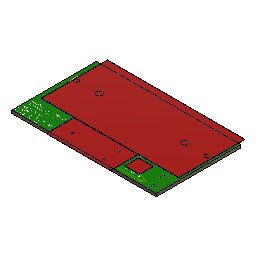
Trashcan Panda v2 v9 (Autodesk Fusion 360 archive; units mm, degrees)
design "Battery-Board"
part number: B2B-PH-SM4-TB(LF)(SN)
part number: HLC-1520A/TP
part number: 2232
Autodesk Fusion 360 part; units mm, degrees
sketch "sketch 305" plane through (0, 0, 0) normal (0, 0, 1) x (1, 0, 0)
  line L0 (0, 0) -> (77.45, 0)
  line L1 (77.45, 0) -> (77.45, 45.39)
  line L2 (77.45, 45.39) -> (0, 45.39)
  line L3 (0, 45.39) -> (0, 0)
extrude "Board" add sketch "sketch 305" along normal blind 1.57 makes body 1 in component "Board"
sketch "sketch 764" plane through (0, 0, 0) normal (0, 0, 1) x (1, 0, 0)
  line L0 (-3.975, -2.624) -> (3.975, -2.624)
  line L1 (3.975, -2.624) -> (3.975, 4.75)
  line L2 (3.975, 4.75) -> (-3.975, 4.75)
  line L3 (-3.975, 4.75) -> (-3.975, -2.624)
extrude "JST_B2B-PH-SM4-TB(LF)(SN)" add sketch "sketch 764" along normal blind 0.1 separate body makes body 2 in component "JST_B2B-PH-SM4-TB(LF)(SN)"
sketch "sketch 1034" plane through (0, 0, 0) normal (0, 0, 1) x (1, 0, 0)
  line L0 (-17.145, -7.4) -> (17.248, -7.4)
  line L1 (17.248, -7.4) -> (17.248, 7.4)
  line L2 (17.248, 7.4) -> (-17.145, 7.4)
  line L3 (-17.145, 7.4) -> (-17.145, -7.4)
extrude "HLC-1520A/TP" add sketch "sketch 1034" along normal blind 0.1 separate body makes body 3 in component "HLC-1520A/TP"
sketch "sketch 1369" plane through (0, 0, 0) normal (0, 0, 1) x (1, 0, 0)
  line L0 (-36.195, -17.78) -> (37.568, -17.78)
  line L1 (37.568, -17.78) -> (37.568, 17.78)
  line L2 (37.568, 17.78) -> (-36.195, 17.78)
  line L3 (-36.195, 17.78) -> (-36.195, -17.78)
extrude "2232" add sketch "sketch 1369" along normal blind 0.1 separate body makes body 4 in component "2232"
sketch "sketch 1173" plane through (0, 0, 0) normal (0, 0, 1) x (1, 0, 0)
  circle A0 centre (70.993, 8.763) radius 0.175
  circle A1 centre (72.644, 3.556) radius 0.175
  circle A2 centre (74.168, 3.556) radius 0.175
  circle A3 centre (72.644, 2.286) radius 0.175
  circle A4 centre (73.787, 10.668) radius 0.175
  circle A5 centre (70.993, 10.668) radius 0.175
  circle A6 centre (3.683, 31.115) radius 1.092
  circle A7 centre (73.533, 31.115) radius 1.092
  circle A8 centre (15.748, 31.115) radius 1.5875
  circle A9 centre (61.468, 31.115) radius 1.5875
  circle A10 centre (26.838, 5.715) radius 0.4
  circle A11 centre (47.838, 9.465) radius 0.4
  circle A12 centre (47.838, 1.965) radius 0.4
extrude "Extrude3" cut sketch "sketch 1173" along normal blind 1.57 bodies 1 in component "Board"
component "PCB Component" placed x (1, 0, 0) y (0, 1, 0) z (0, 0, 1) at (0, 0, 0)
component "Board" placed x (1, 0, 0) y (0, 1, 0) z (0, 0, 1) at (0, 0, 0) in component "PCB Component"
component "JST_B2B-PH-SM4-TB(LF)(SN)" placed x (1, 0, 0) y (0, 1, 0) z (0, 0, 1) at (60.198, 6.985, 1.57) in component "PCB Component"
component "HLC-1520A/TP" placed x (1, 0, 0) y (0, 1, 0) z (0, 0, 1) at (37.338, 5.715, 1.57) in component "PCB Component"
component "2232" placed x (1, 0, 0) y (0, 1, 0) z (0, 0, 1) at (38.608, 31.115, 1.57) in component "PCB Component"
named bodies: "Board", "JST_B2B-PH-SM4-TB(LF)(SN)", "HLC-1520A/TP", "2232"

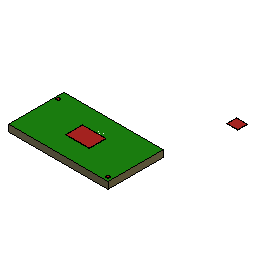
design "Sensor Breakout"
part number: FIDUCIALUFIDUCIAL
part number: 0.1uF
part number: OSHW-LOGOMINI
part number: VL53L1X
part number: 10k
part number: BM06B-SRSS-TBT(LF)(SN)
part number: LIS3DH
part number: 100k
part number: BSS215P
Autodesk Fusion 360 part; units mm, degrees
sketch "sketch 305" plane through (0, 0, 0) normal (0, 0, 1) x (1, 0, 0)
  line L0 (0, 0) -> (0, 12.7)
  line L1 (0, 12.7) -> (22.86, 12.7)
  line L2 (22.86, 12.7) -> (22.86, 0)
  line L3 (22.86, 0) -> (0, 0)
extrude "Board" add sketch "sketch 305" along normal blind 1.57 makes body 1 in component "Board"
sketch "sketch 499" plane through (0, 0, 0) normal (0, 0, 1) x (1, 0, 0)
  line L0 (-0.3175, -0.3175) -> (0.3175, -0.3175)
  line L1 (0.3175, -0.3175) -> (0.3175, 0.3175)
  line L2 (0.3175, 0.3175) -> (-0.3175, 0.3175)
  line L3 (-0.3175, 0.3175) -> (-0.3175, -0.3175)
extrude "MICRO-FIDUCIAL" add sketch "sketch 499" along normal blind 0.1 separate body makes body 2 in component "MICRO-FIDUCIAL"
sketch "sketch 634" plane through (0, 0, 0) normal (0, 0, 1) x (1, 0, 0)
  line L0 (-0.838, -0.47) -> (0.83, -0.47)
  line L1 (0.83, -0.47) -> (0.83, 0.48)
  line L2 (0.83, 0.48) -> (-0.838, 0.48)
  line L3 (-0.838, 0.48) -> (-0.838, -0.47)
extrude "0603" add sketch "sketch 634" along normal blind 0.1 separate body makes body 3 in component "0603"
sketch "sketch 769" plane through (0, 0, 0) normal (0, 0, 1) x (1, 0, 0)
  line L0 (-1.233, -0.993) -> (1.237, -0.993)
  line L1 (1.237, -0.993) -> (1.237, 1.217)
  line L2 (1.237, 1.217) -> (-1.233, 1.217)
  line L3 (-1.233, 1.217) -> (-1.233, -0.993)
extrude "OSHW-LOGO-MINI" add sketch "sketch 769" along normal blind 0.1 separate body makes body 4 in component "OSHW-LOGO-MINI"
sketch "sketch 904" plane through (0, 0, 0) normal (0, 0, 1) x (1, 0, 0)
  line L0 (-2.7, -1.941) -> (2.7, -1.941)
  line L1 (2.7, -1.941) -> (2.7, 1.9)
  line L2 (2.7, 1.9) -> (-2.7, 1.9)
  line L3 (-2.7, 1.9) -> (-2.7, -1.941)
extrude "VL53L1X" add sketch "sketch 904" along normal blind 0.1 separate body makes body 5 in component "VL53L1X"
sketch "sketch 1039" plane through (0, 0, 0) normal (0, 0, 1) x (1, 0, 0)
  line L0 (-0.838, -0.47) -> (0.83, -0.47)
  line L1 (0.83, -0.47) -> (0.83, 0.48)
  line L2 (0.83, 0.48) -> (-0.838, 0.48)
  line L3 (-0.838, 0.48) -> (-0.838, -0.47)
extrude "0603'" add sketch "sketch 1039" along normal blind 0.1 separate body makes body 6 in component "0603 (1)"
sketch "sketch 1174" plane through (0, 0, 0) normal (0, 0, 1) x (1, 0, 0)
  line L0 (-4, -3.031) -> (4, -3.031)
  line L1 (4, -3.031) -> (4, 0.7)
  line L2 (4, 0.7) -> (-4, 0.7)
  line L3 (-4, 0.7) -> (-4, -3.031)
extrude "JST_BM06B-SRSS-TB(LF)(SN)" add sketch "sketch 1174" along normal blind 0.1 separate body makes body 7 in component "JST_BM06B-SRSS-TB(LF)(SN)"
sketch "sketch 1309" plane through (0, 0, 0) normal (0, 0, 1) x (1, 0, 0)
  line L0 (-2.003, -1.5) -> (1.5, -1.5)
  line L1 (1.5, -1.5) -> (1.5, 1.5)
  line L2 (1.5, 1.5) -> (-2.003, 1.5)
  line L3 (-2.003, 1.5) -> (-2.003, -1.5)
extrude "PQFN50P300X300X100-16N" add sketch "sketch 1309" along normal blind 0.1 separate body makes body 8 in component "PQFN50P300X300X100-16N"
sketch "sketch 1444" plane through (0, 0, 0) normal (0, 0, 1) x (1, 0, 0)
  line L0 (-2.2, -1.1) -> (2.2, -1.1)
  line L1 (2.2, -1.1) -> (2.2, 1.1)
  line L2 (2.2, 1.1) -> (-2.2, 1.1)
  line L3 (-2.2, 1.1) -> (-2.2, -1.1)
extrude "C1206" add sketch "sketch 1444" along normal blind 0.1 separate body makes body 9 in component "C1206"
sketch "sketch 1579" plane through (0, 0, 0) normal (0, 0, 1) x (1, 0, 0)
  line L0 (-1.3, 0.6) -> (1.3, 0.6)
  line L1 (1.3, 0.6) -> (1.3, -0.6)
  line L2 (1.3, -0.6) -> (-1.3, -0.6)
  line L3 (-1.3, -0.6) -> (-1.3, 0.6)
extrude "0805" add sketch "sketch 1579" along normal blind 1.645 separate body makes body 10 in component "0805"
sketch "sketch 1714" plane through (0, 0, 0) normal (0, 0, 1) x (1, 0, 0)
  line L0 (-1.651, -2.642) -> (1.651, -2.642)
  line L1 (1.651, -2.642) -> (1.651, 1.321)
  line L2 (1.651, 1.321) -> (-1.651, 1.321)
  line L3 (-1.651, 1.321) -> (-1.651, -2.642)
extrude "SOT-23_3L_ONS-M" add sketch "sketch 1714" along normal blind 0.1 separate body makes body 11 in component "SOT-23_3L_ONS-M"
component "PCB Component" placed x (1, 0, 0) y (0, 1, 0) z (0, 0, 1) at (0, 0, 0)
component "Board" placed x (1, 0, 0) y (0, 1, 0) z (0, 0, 1) at (0, 0, 0) in component "PCB Component"
component "MICRO-FIDUCIAL" placed x (1, 0, 0) y (0, 1, 0) z (0, 0, 1) at (21.971, 0.889, 1.57) in component "PCB Component"
component "MICRO-FIDUCIAL" placed x (1, 0, 0) y (0, 1, 0) z (0, 0, 1) at (0.762, 10.668, 1.57) in component "PCB Component"
component "MICRO-FIDUCIAL" placed x (-1, 0, 0) y (0, 1, 0) z (0, 0, -1) at (0.762, 10.668, 0) in component "PCB Component"
component "MICRO-FIDUCIAL" placed x (-1, 0, 0) y (0, 1, 0) z (0, 0, -1) at (21.971, 0.889, 0) in component "PCB Component"
component "0603" placed x (0, -1, 0) y (-1, 0, 0) z (0, 0, -1) at (15.621, 6.35, 0) in component "PCB Component"
component "OSHW-LOGO-MINI" placed x (-1, 0, 0) y (0, 1, 0) z (0, 0, -1) at (24.638, 27.813, 0) in component "PCB Component"
component "VL53L1X" placed x (1, 0, 0) y (0, 1, 0) z (0, 0, 1) at (11.43, 6.35, 1.57) in component "PCB Component"
component "0603 (1)" placed x (0, 1, 0) y (1, 0, 0) z (0, 0, -1) at (11.303, 6.35, 0) in component "PCB Component"
component "JST_BM06B-SRSS-TB(LF)(SN)" placed x (0, -1, 0) y (-1, 0, 0) z (0, 0, -1) at (2.921, 6.35, 0) in component "PCB Component"
component "PQFN50P300X300X100-16N" placed x (0, -1, 0) y (-1, 0, 0) z (0, 0, -1) at (19.05, 6.35, 0) in component "PCB Component"
component "C1206" placed x (0, -1, 0) y (-1, 0, 0) z (0, 0, -1) at (13.462, 6.35, 0) in component "PCB Component"
component "0805" placed x (-1, 0, 0) y (0, 1, 0) z (0, 0, -1) at (6.35, 2.54, 0) in component "PCB Component"
component "SOT-23_3L_ONS-M" placed x (-1, 0, 0) y (0, 1, 0) z (0, 0, -1) at (6.35, 5.08, 0) in component "PCB Component"
named bodies: "Board", "MICRO-FIDUCIAL", "0603", "OSHW-LOGO-MINI", "VL53L1X", "JST_BM06B-SRSS-TB(LF)(SN)", "PQFN50P300X300X100-16N", "C1206", "0805", "SOT-23_3L_ONS-M"

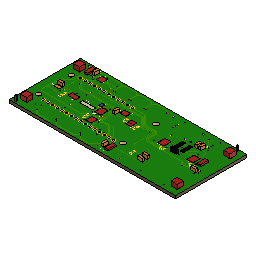
design "Carrier Board"
part number: 0.1uF
part number: D5V0L4B5TS
part number: 4.7k
part number: 100k
part number: TMP36GRTZ
part number: FIDUCIALUFIDUCIAL
part number: STAND-OFF
part number: 6V/0.5A
part number: 470uF
part number: Particle Boron / Xenon / Argon
part number: MF-SW-TACT-6MM
part number: BAT42
part number: JUMPER-SMT_2_NO_SILK
part number: 6.2V/500mW
part number: CL-SB-12B-01T
part number: BM04B-SRSS-TBT(LF)(SN)
part number: BM06B-SRSS-TBT(LF)(SN)
part number: AB1805-T3
part number: XC6215B332MR-G
part number: BSS138
part number: MB85RC64TASON8
part number: B2B-PH-SM4-TB(LF)(SN)
part number: GRM21A5C2D470JW01D
part number: BSS215P
part number: SSPT7F-7PF20-R
Autodesk Fusion 360 part; units mm, degrees
sketch "sketch 305" plane through (0, 0, 0) normal (0, 0, 1) x (1, 0, 0)
  line L0 (0, 0) -> (89.967, 0)
  line L1 (89.967, 0) -> (89.967, 38.608)
  line L2 (89.967, 38.608) -> (0, 38.608)
  line L3 (0, 38.608) -> (0, 0)
extrude "Board" add sketch "sketch 305" along normal blind 1.5723 makes body 1 in component "Board"
sketch "sketch 1247" plane through (0, 0, 0) normal (0, 0, 1) x (1, 0, 0)
  line L0 (-0.3, -0.6) -> (0.3, -0.6)
  line L1 (0.3, -0.6) -> (0.3, 0.6)
  line L2 (0.3, 0.6) -> (-0.3, 0.6)
  line L3 (-0.3, 0.6) -> (-0.3, -0.6)
extrude "0805@1" add sketch "sketch 1247" along normal blind 0.1 separate body makes body 2 in component "0805@1"
sketch "sketch 1382" plane through (0, 0, 0) normal (0, 0, 1) x (1, 0, 0)
  line L0 (-1.727, -1.5) -> (1.4, -1.5)
  line L1 (1.4, -1.5) -> (1.4, 1.5)
  line L2 (1.4, 1.5) -> (-1.727, 1.5)
  line L3 (-1.727, 1.5) -> (-1.727, -1.5)
extrude "SOT-23-5" add sketch "sketch 1382" along normal blind 0.1 separate body makes body 3 in component "SOT-23-5"
sketch "sketch 1517" plane through (0, 0, 0) normal (0, 0, 1) x (1, 0, 0)
  line L0 (-1.5, -0.8) -> (1.5, -0.8)
  line L1 (1.5, -0.8) -> (1.5, 0.8)
  line L2 (1.5, 0.8) -> (-1.5, 0.8)
  line L3 (-1.5, 0.8) -> (-1.5, -0.8)
extrude "0805" add sketch "sketch 1517" along normal blind 0.1 separate body makes body 4 in component "0805"
sketch "sketch 1716" plane through (0, 0, 0) normal (0, 0, 1) x (1, 0, 0)
  line L0 (-1.3, 0.6) -> (1.3, 0.6)
  line L1 (1.3, 0.6) -> (1.3, -0.6)
  line L2 (1.3, -0.6) -> (-1.3, -0.6)
  line L3 (-1.3, -0.6) -> (-1.3, 0.6)
extrude "0805'" add sketch "sketch 1716" along normal blind 1.645 separate body makes body 5 in component "0805 (1)"
sketch "sketch 1851" plane through (0, 0, 0) normal (0, 0, 1) x (1, 0, 0)
  line L0 (-1.499, -1.626) -> (1.499, -1.626)
  line L1 (1.499, -1.626) -> (1.499, 1.804)
  line L2 (1.499, 1.804) -> (-1.499, 1.804)
  line L3 (-1.499, 1.804) -> (-1.499, -1.626)
extrude "RJ_5_ADI" add sketch "sketch 1851" along normal blind 0.1 separate body makes body 6 in component "RJ_5_ADI"
sketch "sketch 1994" plane through (0, 0, 0) normal (0, 0, 1) x (1, 0, 0)
  line L0 (-0.3175, 0.3175) -> (0.3175, 0.3175)
  line L1 (0.3175, 0.3175) -> (0.3175, -0.3175)
  line L2 (0.3175, -0.3175) -> (-0.3175, -0.3175)
  line L3 (-0.3175, -0.3175) -> (-0.3175, 0.3175)
extrude "FIDUCIAL-MICRO" add sketch "sketch 1994" along normal blind 2.613 separate body makes body 7 in component "FIDUCIAL-MICRO"
sketch "sketch 2153" plane through (0, 0, 0) normal (0, 0, 1) x (1, 0, 0)
  line L0 (-1.6535, 1.651) -> (1.6535, 1.651)
  line L1 (1.6535, 1.651) -> (1.6535, -1.651)
  line L2 (1.6535, -1.651) -> (-1.6535, -1.651)
  line L3 (-1.6535, -1.651) -> (-1.6535, 1.651)
extrude "STAND-OFF" add sketch "sketch 2153" along normal blind 2.293 separate body makes body 8 in component "STAND-OFF"
sketch "sketch 2304" plane through (0, 0, 0) normal (0, 0, 1) x (1, 0, 0)
  line L0 (-2.2, 0.9) -> (2.2, 0.9)
  line L1 (2.2, 0.9) -> (2.2, -0.9)
  line L2 (2.2, -0.9) -> (-2.2, -0.9)
  line L3 (-2.2, -0.9) -> (-2.2, 0.9)
extrude "1206" add sketch "sketch 2304" along normal blind 0.866 separate body makes body 9 in component "1206"
sketch "sketch 2439" plane through (0, 0, 0) normal (0, 0, 1) x (1, 0, 0)
  line L0 (-2.481, -1.97) -> (2.481, -1.97)
  line L1 (2.481, -1.97) -> (2.481, 2.481)
  line L2 (2.481, 2.481) -> (-2.481, 2.481)
  line L3 (-2.481, 2.481) -> (-2.481, -1.97)
extrude "OSHW-LOGO-M" add sketch "sketch 2439" along normal blind 0.1 separate body makes body 10 in component "OSHW-LOGO-M"
sketch "sketch 2574" plane through (0, 0, 0) normal (0, 0, 1) x (1, 0, 0)
  line L0 (-5.15, -5.15) -> (5.15, -5.15)
  line L1 (5.15, -5.15) -> (5.15, 5.15)
  line L2 (5.15, 5.15) -> (-5.15, 5.15)
  line L3 (-5.15, 5.15) -> (-5.15, -5.15)
extrude "CP10MM" add sketch "sketch 2574" along normal blind 0.1 separate body makes body 11 in component "CP10MM"
sketch "sketch 2709" plane through (0, 0, 0) normal (0, 0, 1) x (1, 0, 0)
  line L0 (0, 0) -> (22.86, 0)
  line L1 (22.86, 0) -> (22.86, 52.07)
  line L2 (22.86, 52.07) -> (0, 52.07)
  line L3 (0, 52.07) -> (0, 0)
extrude "PARTICLE-DEVICES_BORON" add sketch "sketch 2709" along normal blind 0.1 separate body makes body 12 in component "PARTICLE-DEVICES_BORON"
sketch "sketch 2844" plane through (0, 0, 0) normal (0, 0, 1) x (1, 0, 0)
  line L0 (-5.2, -3.4) -> (5.2, -3.4)
  line L1 (5.2, -3.4) -> (5.2, 3.4)
  line L2 (5.2, 3.4) -> (-5.2, 3.4)
  line L3 (-5.2, 3.4) -> (-5.2, -3.4)
extrude "TACT6MM" add sketch "sketch 2844" along normal blind 0.1 separate body makes body 13 in component "TACT6MM"
sketch "sketch 2987" plane through (0, 0, 0) normal (0, 0, 1) x (1, 0, 0)
  line L0 (-2.8, -0.85) -> (2.4, -0.85)
  line L1 (2.4, -0.85) -> (2.4, 0.85)
  line L2 (2.4, 0.85) -> (-2.8, 0.85)
  line L3 (-2.8, 0.85) -> (-2.8, -0.85)
extrude "SOD-123" add sketch "sketch 2987" along normal blind 0.1 separate body makes body 14 in component "SOD-123"
sketch "sketch 3122" plane through (0, 0, 0) normal (0, 0, 1) x (1, 0, 0)
  line L0 (-0.7239, 0.635) -> (0.7239, 0.635)
  line L1 (0.7239, 0.635) -> (0.7239, -0.635)
  line L2 (0.7239, -0.635) -> (-0.7239, -0.635)
  line L3 (-0.7239, -0.635) -> (-0.7239, 0.635)
extrude "SMT-JUMPER_2_NO_SILK" add sketch "sketch 3122" along normal blind 1.962 separate body makes body 15 in component "SMT-JUMPER_2_NO_SILK"
sketch "sketch 3257" plane through (0, 0, 0) normal (0, 0, 1) x (1, 0, 0)
  line L0 (-1.65, 0.55) -> (1.65, 0.55)
  line L1 (1.65, 0.55) -> (1.65, -0.55)
  line L2 (1.65, -0.55) -> (-1.65, -0.55)
  line L3 (-1.65, -0.55) -> (-1.65, 0.55)
extrude "PANASONIC_SMINI2-F5-B" add sketch "sketch 3257" along normal blind 2.031 separate body makes body 16 in component "PANASONIC_SMINI2-F5-B"
sketch "sketch 3392" plane through (0, 0, 0) normal (0, 0, 1) x (1, 0, 0)
  line L0 (-4.25, -1.75) -> (4.25, -1.75)
  line L1 (4.25, -1.75) -> (4.25, 1.75)
  line L2 (4.25, 1.75) -> (-4.25, 1.75)
  line L3 (-4.25, 1.75) -> (-4.25, -1.75)
extrude "CL-SB-12B" add sketch "sketch 3392" along normal blind 0.1 separate body makes body 17 in component "CL-SB-12B"
sketch "sketch 3551" plane through (0, 0, 0) normal (0, 0, 1) x (1, 0, 0)
  line L0 (-3, -3.16) -> (3, -3.16)
  line L1 (3, -3.16) -> (3, 0.7)
  line L2 (3, 0.7) -> (-3, 0.7)
  line L3 (-3, 0.7) -> (-3, -3.16)
extrude "CONN_BM04B-SRSS-TBT(LF)(SN)" add sketch "sketch 3551" along normal blind 0.1 separate body makes body 18 in component "CONN_BM04B-SRSS-TBT(LF)(SN)"
sketch "sketch 3702" plane through (0, 0, 0) normal (0, 0, 1) x (1, 0, 0)
  line L0 (-4, -3.031) -> (4, -3.031)
  line L1 (4, -3.031) -> (4, 0.7)
  line L2 (4, 0.7) -> (-4, 0.7)
  line L3 (-4, 0.7) -> (-4, -3.031)
extrude "JST_BM06B-SRSS-TB(LF)(SN)" add sketch "sketch 3702" along normal blind 0.1 separate body makes body 19 in component "JST_BM06B-SRSS-TB(LF)(SN)"
sketch "sketch 3837" plane through (0, 0, 0) normal (0, 0, 1) x (1, 0, 0)
  line L0 (-1.651, -1.651) -> (2.35, -1.651)
  line L1 (2.35, -1.651) -> (2.35, 1.651)
  line L2 (2.35, 1.651) -> (-1.651, 1.651)
  line L3 (-1.651, 1.651) -> (-1.651, -1.651)
extrude "QFN_16_ABR" add sketch "sketch 3837" along normal blind 0.1 separate body makes body 20 in component "QFN_16_ABR"
sketch "sketch 3972" plane through (0, 0, 0) normal (0, 0, 1) x (1, 0, 0)
  line L0 (-1.397, -1.575) -> (1.397, -1.575)
  line L1 (1.397, -1.575) -> (1.397, 1.575)
  line L2 (1.397, 1.575) -> (-1.397, 1.575)
  line L3 (-1.397, 1.575) -> (-1.397, -1.575)
extrude "SOT-25_TOR" add sketch "sketch 3972" along normal blind 0.1 separate body makes body 21 in component "SOT-25_TOR"
sketch "sketch 4107" plane through (0, 0, 0) normal (0, 0, 1) x (1, 0, 0)
  line L0 (-1.651, -1.321) -> (1.651, -1.321)
  line L1 (1.651, -1.321) -> (1.651, 1.321)
  line L2 (1.651, 1.321) -> (-1.651, 1.321)
  line L3 (-1.651, 1.321) -> (-1.651, -1.321)
extrude "SOT-23_3L_ONS" add sketch "sketch 4107" along normal blind 0.1 separate body makes body 22 in component "SOT-23_3L_ONS"
sketch "sketch 4242" plane through (0, 0, 0) normal (0, 0, 1) x (1, 0, 0)
  line L0 (-2.6, -1.199) -> (1.54, -1.199)
  line L1 (1.54, -1.199) -> (1.54, 1.199)
  line L2 (1.54, 1.199) -> (-2.6, 1.199)
  line L3 (-2.6, 1.199) -> (-2.6, -1.199)
extrude "SON50P200X300X75-9N" add sketch "sketch 4242" along normal blind 0.1 separate body makes body 23 in component "SON50P200X300X75-9N"
sketch "sketch 4385" plane through (0, 0, 0) normal (0, 0, 1) x (1, 0, 0)
  line L0 (-3.975, -2.624) -> (3.975, -2.624)
  line L1 (3.975, -2.624) -> (3.975, 4.75)
  line L2 (3.975, 4.75) -> (-3.975, 4.75)
  line L3 (-3.975, 4.75) -> (-3.975, -2.624)
extrude "JST_B2B-PH-SM4-TB(LF)(SN)" add sketch "sketch 4385" along normal blind 0.1 separate body makes body 24 in component "JST_B2B-PH-SM4-TB(LF)(SN)"
sketch "sketch 4520" plane through (0, 0, 0) normal (0, 0, 1) x (1, 0, 0)
  line L0 (-1.1, -0.72) -> (1.1, -0.72)
  line L1 (1.1, -0.72) -> (1.1, 0.72)
  line L2 (1.1, 0.72) -> (-1.1, 0.72)
  line L3 (-1.1, 0.72) -> (-1.1, -0.72)
extrude "CAPC2012X100N" add sketch "sketch 4520" along normal blind 0.1 separate body makes body 25 in component "CAPC2012X100N"
sketch "sketch 4663" plane through (0, 0, 0) normal (0, 0, 1) x (1, 0, 0)
  line L0 (-1.651, -2.642) -> (1.651, -2.642)
  line L1 (1.651, -2.642) -> (1.651, 1.321)
  line L2 (1.651, 1.321) -> (-1.651, 1.321)
  line L3 (-1.651, 1.321) -> (-1.651, -2.642)
extrude "SOT-23_3L_ONS-M" add sketch "sketch 4663" along normal blind 0.1 separate body makes body 26 in component "SOT-23_3L_ONS-M"
sketch "sketch 4798" plane through (0, 0, 0) normal (0, 0, 1) x (1, 0, 0)
  line L0 (-0.864, -3.505) -> (0.864, -3.505)
  line L1 (0.864, -3.505) -> (0.864, 3.505)
  line L2 (0.864, 3.505) -> (-0.864, 3.505)
  line L3 (-0.864, 3.505) -> (-0.864, -3.505)
extrude "SSP-T7-F_EPS" add sketch "sketch 4798" along normal blind 0.1 separate body makes body 27 in component "SSP-T7-F_EPS"
sketch "sketch 412" plane through (0, 0, 0) normal (0, 0, 1) x (1, 0, 0)
  circle A0 centre (18.796, 13.97) radius 0.175
  circle A1 centre (18.796, 11.43) radius 0.175
  circle A2 centre (44.196, 21.844) radius 0.175
  circle A3 centre (18.796, 23.114) radius 0.175
  circle A4 centre (28.448, 16.764) radius 0.175
  circle A5 centre (76.454, 33.782) radius 0.175
  circle A6 centre (77.47, 36.83) radius 0.175
  circle A7 centre (57.404, 33.782) radius 0.175
  circle A8 centre (57.404, 31.242) radius 0.175
  circle A9 centre (85.598, 16.764) radius 0.175
  circle A10 centre (34.544, 13.716) radius 0.175
  circle A11 centre (29.464, 10.922) radius 0.175
  circle A12 centre (64.77, 20.066) radius 0.175
  circle A13 centre (84.074, 18.288) radius 0.175
  circle A14 centre (84.582, 15.24) radius 0.175
  circle A15 centre (85.09, 18.288) radius 0.175
  circle A16 centre (76.454, 32.512) radius 0.175
  circle A17 centre (57.404, 32.512) radius 0.175
  circle A18 centre (38.608, 10.414) radius 0.175
  circle A19 centre (40.894, 10.414) radius 0.175
  circle A20 centre (39.878, 7.62) radius 0.175
  circle A21 centre (11.938, 33.274) radius 0.175
  circle A22 centre (10.922, 33.274) radius 0.175
  circle A23 centre (5.842, 37.338) radius 0.175
  circle A24 centre (52.578, 36.83) radius 0.175
  circle A25 centre (58.42, 36.83) radius 0.175
  circle A26 centre (76.454, 31.242) radius 0.175
  circle A27 centre (77.47, 29.972) radius 0.175
  circle A28 centre (41.656, 32.385) radius 0.175
  circle A29 centre (58.166, 20.066) radius 0.175
  circle A30 centre (31.75, 22.606) radius 0.175
  circle A31 centre (9.144, 5.08) radius 0.175
  circle A32 centre (45.466, 2.286) radius 0.175
  circle A33 centre (57.404, 2.286) radius 0.175
  circle A34 centre (68.834, 2.286) radius 0.175
  circle A35 centre (81.534, 2.286) radius 0.175
  circle A36 centre (52.578, 35.814) radius 0.175
  circle A37 centre (13.208, 32.258) radius 0.175
  circle A38 centre (33.02, 17.018) radius 0.175
  circle A39 centre (9.652, 18.034) radius 0.175
  circle A40 centre (33.528, 32.385) radius 0.175
  circle A41 centre (25.146, 32.258) radius 0.175
  circle A42 centre (18.796, 25.654) radius 0.175
  circle A43 centre (15.494, 21.082) radius 0.175
  circle A44 centre (11.176, 6.35) radius 0.175
  circle A45 centre (21.844, 3.556) radius 0.175
  circle A46 centre (34.798, 3.556) radius 0.175
  circle A47 centre (80.518, 20.066) radius 0.175
  circle A48 centre (22.106, 32.273) radius 0.175
  circle A49 centre (9.906, 19.558) radius 0.175
  circle A50 centre (11.76, 26.416) radius 0.175
  circle A51 centre (23.106, 35.321) radius 0.175
  circle A52 centre (16.51, 36.576) radius 0.175
  circle A53 centre (12.192, 2.794) radius 0.175
  circle A54 centre (22.86, 2.794) radius 0.175
  circle A55 centre (35.814, 2.794) radius 0.175
  circle A56 centre (61.558, 8.382) radius 0.175
  circle A57 centre (30.226, 21.59) radius 0.175
  circle A58 centre (36.322, 26.67) radius 0.175
  circle A59 centre (77.47, 16.002) radius 0.175
  circle A60 centre (48.768, 36.322) radius 0.175
  circle A61 centre (32.504, 32.398) radius 0.175
  circle A62 centre (40.632, 32.398) radius 0.175
  circle A63 centre (24.106, 32.273) radius 0.175
  circle A64 centre (69.088, 24.384) radius 0.175
  circle A65 centre (60.452, 27.178) radius 0.175
  circle A66 centre (53.086, 22.863) radius 0.175
  circle A67 centre (66.04, 28.956) radius 0.175
  circle A68 centre (72.644, 35.306) radius 0.175
  circle A69 centre (76.708, 25.4) radius 0.175
  circle A70 centre (29.018, 21.274) radius 0.175
  circle A71 centre (30.572, 16.586) radius 0.175
  circle A72 centre (71.628, 20.066) radius 0.175
  circle A73 centre (72.644, 32.512) radius 0.175
  circle A74 centre (4.445, 33.604) radius 1.651
  circle A75 centre (85.852, 33.604) radius 1.651
  circle A76 centre (85.852, 5.029) radius 1.651
  circle A77 centre (4.445, 5.029) radius 1.651
  circle A78 centre (47.32, 9.22) radius 0.508
  circle A79 centre (44.78, 9.22) radius 0.508
  circle A80 centre (42.24, 9.22) radius 0.508
  circle A81 centre (39.7, 9.22) radius 0.508
  circle A82 centre (37.16, 9.22) radius 0.508
  circle A83 centre (34.62, 9.22) radius 0.508
  circle A84 centre (32.08, 9.22) radius 0.508
  circle A85 centre (29.54, 9.22) radius 0.508
  circle A86 centre (27, 9.22) radius 0.508
  circle A87 centre (24.46, 9.22) radius 0.508
  circle A88 centre (21.92, 9.22) radius 0.508
  circle A89 centre (19.38, 9.22) radius 0.508
  circle A90 centre (16.84, 9.22) radius 0.508
  circle A91 centre (14.3, 9.22) radius 0.508
  circle A92 centre (11.76, 9.22) radius 0.508
  circle A93 centre (9.22, 9.22) radius 0.508
  circle A94 centre (9.22, 29.54) radius 0.508
  circle A95 centre (11.76, 29.54) radius 0.508
  circle A96 centre (14.3, 29.54) radius 0.508
  circle A97 centre (16.84, 29.54) radius 0.508
  circle A98 centre (19.38, 29.54) radius 0.508
  circle A99 centre (21.92, 29.54) radius 0.508
  circle A100 centre (24.46, 29.54) radius 0.508
  circle A101 centre (27, 29.54) radius 0.508
  circle A102 centre (29.54, 29.54) radius 0.508
  circle A103 centre (32.08, 29.54) radius 0.508
  circle A104 centre (34.62, 29.54) radius 0.508
  circle A105 centre (37.16, 29.54) radius 0.508
  circle A106 centre (5.41, 10.49) radius 1.27
  circle A107 centre (5.41, 28.27) radius 1.27
  circle A108 centre (51.13, 28.27) radius 1.27
  circle A109 centre (51.13, 10.49) radius 1.27
  circle A110 centre (68.834, 29.366) radius 0.45
  circle A111 centre (68.834, 36.166) radius 0.45
extrude "Extrude2" cut sketch "sketch 412" along normal blind 1.5723 bodies 1 in component "Board"
component "PCB Component" placed x (1, 0, 0) y (0, 1, 0) z (0, 0, 1) at (0, 0, 0)
component "Board" placed x (1, 0, 0) y (0, 1, 0) z (0, 0, 1) at (0, 0, 0) in component "PCB Component"
component "0805@1" placed x (0, 1, 0) y (-1, 0, 0) z (0, 0, 1) at (11.938, 17.526, 1.5723) in component "PCB Component"
component "0805@1" placed x (0, 1, 0) y (-1, 0, 0) z (0, 0, 1) at (28.448, 12.7, 1.5723) in component "PCB Component"
component "0805@1" placed x (1, 0, 0) y (0, 1, 0) z (0, 0, 1) at (64.008, 18.796, 1.5723) in component "PCB Component"
component "0805@1" placed x (1, 0, 0) y (0, 1, 0) z (0, 0, 1) at (79.756, 18.796, 1.5723) in component "PCB Component"
component "0805@1" placed x (0, -1, 0) y (1, 0, 0) z (0, 0, 1) at (57.912, 8.89, 1.5723) in component "PCB Component"
component "0805@1" placed x (0, 1, 0) y (-1, 0, 0) z (0, 0, 1) at (47.498, 20.828, 1.5723) in component "PCB Component"
component "0805@1" placed x (0, -1, 0) y (1, 0, 0) z (0, 0, 1) at (41.148, 21.844, 1.5723) in component "PCB Component"
component "SOT-23-5" placed x (0, -1, 0) y (1, 0, 0) z (0, 0, 1) at (15.723, 34.341, 1.5723) in component "PCB Component"
component "0805" placed x (-1, 0, 0) y (0, -1, 0) z (0, 0, 1) at (7.112, 19.304, 1.5723) in component "PCB Component"
component "0805 (1)" placed x (-1, 0, 0) y (0, -1, 0) z (0, 0, 1) at (7.112, 21.082, 1.5723) in component "PCB Component"
component "0805 (1)" placed x (-1, 0, 0) y (0, -1, 0) z (0, 0, 1) at (83.312, 16.764, 1.5723) in component "PCB Component"
component "0805 (1)" placed x (0, 1, 0) y (-1, 0, 0) z (0, 0, 1) at (47.142, 4.547, 1.5723) in component "PCB Component"
component "0805 (1)" placed x (-1, 0, 0) y (0, -1, 0) z (0, 0, 1) at (64.008, 7.366, 1.5723) in component "PCB Component"
component "0805 (1)" placed x (1, 0, 0) y (0, 1, 0) z (0, 0, 1) at (64.008, 9.906, 1.5723) in component "PCB Component"
component "0805 (1)" placed x (0, 1, 0) y (-1, 0, 0) z (0, 0, 1) at (11.43, 35.56, 1.5723) in component "PCB Component"
component "0805 (1)" placed x (0, 1, 0) y (-1, 0, 0) z (0, 0, 1) at (73.152, 29.21, 1.5723) in component "PCB Component"
component "0805 (1)" placed x (0, -1, 0) y (1, 0, 0) z (0, 0, 1) at (35.052, 22.86, 1.5723) in component "PCB Component"
component "0805 (1)" placed x (0, 1, 0) y (-1, 0, 0) z (0, 0, 1) at (75.184, 29.21, 1.5723) in component "PCB Component"
component "RJ_5_ADI" placed x (1, 0, 0) y (0, 1, 0) z (0, 0, 1) at (31.75, 12.7, 1.5723) in component "PCB Component"
component "FIDUCIAL-MICRO" placed x (1, 0, 0) y (0, 1, 0) z (0, 0, 1) at (85.7, 37.77, 1.5723) in component "PCB Component"
component "FIDUCIAL-MICRO" placed x (1, 0, 0) y (0, 1, 0) z (0, 0, 1) at (2.362, 1.372, 1.5723) in component "PCB Component"
component "STAND-OFF" placed x (1, 0, 0) y (0, 1, 0) z (0, 0, 1) at (4.445, 33.604, 1.5723) in component "PCB Component"
component "STAND-OFF" placed x (1, 0, 0) y (0, 1, 0) z (0, 0, 1) at (85.852, 33.604, 1.5723) in component "PCB Component"
component "STAND-OFF" placed x (0, 1, 0) y (-1, 0, 0) z (0, 0, 1) at (85.852, 5.029, 1.5723) in component "PCB Component"
component "STAND-OFF" placed x (1, 0, 0) y (0, 1, 0) z (0, 0, 1) at (4.445, 5.029, 1.5723) in component "PCB Component"
component "1206" placed x (0, -1, 0) y (1, 0, 0) z (0, 0, 1) at (82.296, 22.352, 1.5723) in component "PCB Component"
component "1206" placed x (0, -1, 0) y (1, 0, 0) z (0, 0, 1) at (49.987, 4.775, 1.5723) in component "PCB Component"
component "1206" placed x (0, 1, 0) y (-1, 0, 0) z (0, 0, 1) at (8.89, 34.798, 1.5723) in component "PCB Component"
component "OSHW-LOGO-M" placed x (0, 1, 0) y (1, 0, 0) z (0, 0, -1) at (86.157, 11.557, 0) in component "PCB Component"
component "CP10MM" placed x (1, 0, 0) y (0, -1, 0) z (0, 0, -1) at (77.47, 8.636, 0) in component "PCB Component"
component "PARTICLE-DEVICES_BORON" placed x (0, 1, 0) y (1, 0, 0) z (0, 0, -1) at (2.87, 7.95, 0) in component "PCB Component"
component "TACT6MM" placed x (0, -1, 0) y (-1, 0, 0) z (0, 0, -1) at (64.008, 8.128, 0) in component "PCB Component"
component "SOD-123" placed x (0, -1, 0) y (1, 0, 0) z (0, 0, 1) at (67.31, 24.638, 1.5723) in component "PCB Component"
component "SOD-123" placed x (0, -1, 0) y (1, 0, 0) z (0, 0, 1) at (71.12, 24.638, 1.5723) in component "PCB Component"
component "SMT-JUMPER_2_NO_SILK" placed x (0, -1, 0) y (-1, 0, 0) z (0, 0, -1) at (73.66, 21.082, 0) in component "PCB Component"
component "PANASONIC_SMINI2-F5-B" placed x (1, 0, 0) y (0, 1, 0) z (0, 0, 1) at (69.342, 20.066, 1.5723) in component "PCB Component"
component "CL-SB-12B" placed x (0, -1, 0) y (-1, 0, 0) z (0, 0, -1) at (68.834, 32.766, 0) in component "PCB Component"
component "CONN_BM04B-SRSS-TBT(LF)(SN)" placed x (-1, 0, 0) y (0, 1, 0) z (0, 0, -1) at (48.26, 36.322, 0) in component "PCB Component"
component "CONN_BM04B-SRSS-TBT(LF)(SN)" placed x (1, 0, 0) y (0, -1, 0) z (0, 0, -1) at (12.7, 2.54, 0) in component "PCB Component"
component "CONN_BM04B-SRSS-TBT(LF)(SN)" placed x (-1, 0, 0) y (0, 1, 0) z (0, 0, -1) at (40.132, 36.322, 0) in component "PCB Component"
component "CONN_BM04B-SRSS-TBT(LF)(SN)" placed x (-1, 0, 0) y (0, 1, 0) z (0, 0, -1) at (32.004, 36.322, 0) in component "PCB Component"
component "JST_BM06B-SRSS-TB(LF)(SN)" placed x (-1, 0, 0) y (0, 1, 0) z (0, 0, -1) at (22.606, 36.322, 0) in component "PCB Component"
component "JST_BM06B-SRSS-TB(LF)(SN)" placed x (1, 0, 0) y (0, -1, 0) z (0, 0, -1) at (24.384, 2.54, 0) in component "PCB Component"
component "JST_BM06B-SRSS-TB(LF)(SN)" placed x (1, 0, 0) y (0, -1, 0) z (0, 0, -1) at (37.338, 2.54, 0) in component "PCB Component"
component "QFN_16_ABR" placed x (0, 1, 0) y (-1, 0, 0) z (0, 0, 1) at (30.48, 19.05, 1.5723) in component "PCB Component"
component "SOT-25_TOR" placed x (-1, 0, 0) y (0, -1, 0) z (0, 0, 1) at (44.196, 21.844, 1.5723) in component "PCB Component"
component "SOT-23_3L_ONS" placed x (1, 0, 0) y (0, 1, 0) z (0, 0, 1) at (37.846, 24.892, 1.5723) in component "PCB Component"
component "SON50P200X300X75-9N" placed x (-1, 0, 0) y (0, -1, 0) z (0, 0, 1) at (15.494, 19.05, 1.5723) in component "PCB Component"
component "JST_B2B-PH-SM4-TB(LF)(SN)" placed x (-1, 0, 0) y (0, 1, 0) z (0, 0, -1) at (59.436, 33.528, 0) in component "PCB Component"
component "JST_B2B-PH-SM4-TB(LF)(SN)" placed x (-1, 0, 0) y (0, 1, 0) z (0, 0, -1) at (78.486, 33.528, 0) in component "PCB Component"
component "CAPC2012X100N" placed x (0, -1, 0) y (1, 0, 0) z (0, 0, 1) at (27.686, 22.352, 1.5723) in component "PCB Component"
component "SOT-23_3L_ONS-M" placed x (-1, 0, 0) y (0, -1, 0) z (0, 0, 1) at (61.976, 21.336, 1.5723) in component "PCB Component"
component "SOT-23_3L_ONS-M" placed x (-1, 0, 0) y (0, -1, 0) z (0, 0, 1) at (77.724, 21.336, 1.5723) in component "PCB Component"
component "SSP-T7-F_EPS" placed x (0, -1, 0) y (1, 0, 0) z (0, 0, 1) at (23.876, 18.542, 1.5723) in component "PCB Component"
named bodies: "Board", "0805@1", "SOT-23-5", "0805", "RJ_5_ADI", "FIDUCIAL-MICRO", "STAND-OFF", "1206", "OSHW-LOGO-M", "CP10MM", "PARTICLE-DEVICES_BORON", "TACT6MM", "SOD-123", "SMT-JUMPER_2_NO_SILK", "PANASONIC_SMINI2-F5-B", "CL-SB-12B", "CONN_BM04B-SRSS-TBT(LF)(SN)", "JST_BM06B-SRSS-TB(LF)(SN)", "QFN_16_ABR", "SOT-25_TOR", "SOT-23_3L_ONS", "SON50P200X300X75-9N", "JST_B2B-PH-SM4-TB(LF)(SN)", "CAPC2012X100N", "SOT-23_3L_ONS-M", "SSP-T7-F_EPS"
